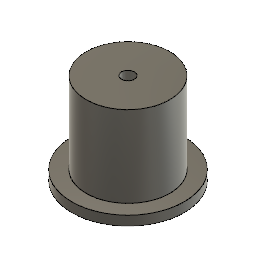
Weight Holder (Autodesk Fusion 360 design; units mm, degrees)
Autodesk Fusion 360 part; units mm, degrees
sketch "Sketch1" plane through (0, 0, 0) normal (0, 1, 0) x (1, 0, 0)
  circle A0 centre (0, 0) radius 13
  circle A1 centre (0, 0) radius 17.5
  circle A2 centre (0, 0) radius 2
  dimension "d1" = 26
  dimension "d2" = 35
  dimension "d7" = 4
  constraint coincident A0.centre A1.centre
  measures "d1" diameter of A0
  measures "d2" diameter of A1
  measures "d7" diameter of A2
extrude "Extrude1" add sketch "Sketch1" along normal blind 25.25 contours A0
extrude "Extrude2" add sketch "Sketch1" against normal blind 3 contours A0 | A1
